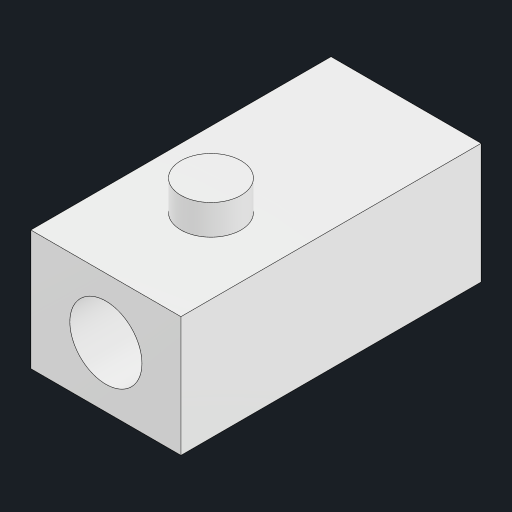
# Autodesk Inventor part: gear_connecotr1_V2
Saved by Autodesk Inventor 2023 (Build 270158000, 158)
## iProperties
Created: 2022-06-15
Part Number: gear_connecotr1_V2
Material: ABS プラスチック
Document SubType Name: Modeling
Designer: legot
Density: 1.06 g/cm^3
Appearance: 滑らか - 白
Mass: 0.227309 g
Surface Area: 3.88253 cm^2
Volume: 0.214443 cm^3
Author: legot
Autodesk Inventor part; units mm, degrees
ref_plane "YZ Plane" through (0, 0, 0) normal (1, 0, 0) x (0, 1, 0)
ref_plane "XZ Plane" through (0, 0, 0) normal (0, 1, 0) x (-1, 0, 0)
ref_plane "XY Plane" through (0, 0, 0) normal (0, 0, 1) x (1, 0, 0)
sketch "スケッチ1" plane through (0, 0, 0) normal (0, 1, 0) x (-1, 0, 0)
  line L0 (2.5, 3.5) -> (-2.5, 3.5)
  line L1 (-2.5, 3.5) -> (-2.5, -6.5)
  line L2 (-2.5, -6.5) -> (2.5, -6.5)
  line L3 (2.5, -6.5) -> (2.5, 3.5)
  point P0 (0, 0)
  point P1 (0, 3.5)
  dimension "d0" = 5
  dimension "d15" = 10
  dimension "d46" = 3.5
  constraints: 8 end point, 2 parallel, 1 horizontal, 1 midpoint, 1 perpendicular, 1 vertical alignment
  measures "d0" distance of L0.start L0.end
  measures "d15" distance of L2.end L0.start
  measures "d46" distance from line of point (0, 0) L0
extrude "押し出し1" add sketch "スケッチ1" along normal mid plane 4
sketch "スケッチ2" plane through (0, 0, 0) normal (0, 1, 0) x (-1, 0, 0)
  circle A0 centre (0, 0) radius 1
  dimension "d3" = 2
  constraints: 1 centre point, 1 coincident
  measures "d3" diameter of A0
extrude "押し出し2" add sketch "スケッチ2" along normal mid plane 6
sketch "スケッチ9" plane through (-2.5, 2, 3.5) normal (0, 0, 1) x (1, 0, 0)
  point P0 (2.5, -2)
  point P1 (2.5, -2)
  constraints: 1 coincident
hole "穴4" at (0, 0, 3.5) direction (0, 0, -1) diameter 2.4 end through all
